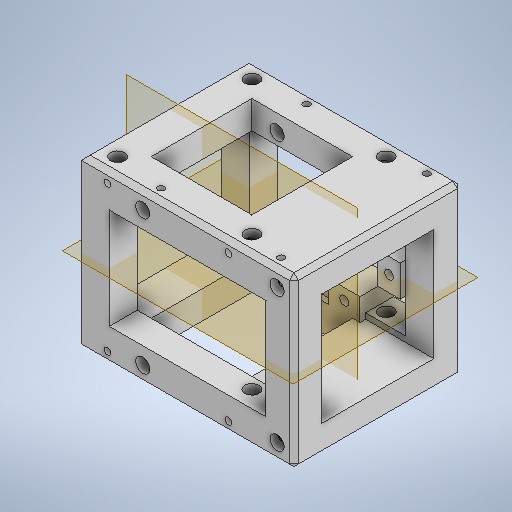
# Autodesk Inventor part: iluminator
Saved by Autodesk Inventor 2025.1 (Build 291241000, 241)
## iProperties
Created: 2024-11-24
Part Number: iluminator
Material: Ogólny
Document SubType Name: Modeling
Designer: zychlix
Density: 1 g/cm^3
Appearance: Domyślna
Author: zychlix
Autodesk Inventor part; units mm, degrees
ref_plane "YZ Plane" through (0, 0, 0) normal (1, 0, 0) x (0, 1, 0)
ref_plane "XZ Plane" through (0, 0, 0) normal (0, 1, 0) x (-1, 0, 0)
ref_plane "XY Plane" through (0, 0, 0) normal (0, 0, 1) x (1, 0, 0)
sketch "Szkic1" plane through (0, 0, 0) normal (0, 0, 1) x (1, 0, 0)
  line L0 (100.1486, 94.401) -> (40.1486, 94.401) construction
  line L1 (40.1486, 94.401) -> (40.1486, 34.401) construction
  line L2 (40.1486, 34.401) -> (100.1486, 34.401) construction
  line L3 (100.1486, 34.401) -> (100.1486, 94.401) construction
  circle A0 centre (100.1486, 94.401) radius 3.175
  circle A1 centre (100.1486, 34.401) radius 3.175
  circle A2 centre (40.1486, 34.401) radius 3.175
  circle A3 centre (40.1486, 94.401) radius 3.175
  line L4 (107.6486, 26.901) -> (12.6486, 26.901)
  line L5 (12.6486, 101.901) -> (107.6486, 101.901)
  line L6 (107.6486, 101.901) -> (107.6486, 26.901)
  line L7 (25.1486, 86.901) -> (95.1486, 86.901)
  line L8 (95.1486, 86.901) -> (95.1486, 41.901)
  line L9 (25.1486, 86.901) -> (25.1486, 41.901)
  line L10 (25.1486, 41.901) -> (95.1486, 41.901)
  line L11 (12.6486, 101.901) -> (12.6486, 26.901)
  point P0 (0, 0)
  point P1 (70.1486, 64.401)
  point P2 (100.1486, 64.401)
  point P3 (70.1486, 94.401)
  point P4 (107.6486, 64.401)
  point P5 (25.1486, 64.401)
  dimension "d0" = 60
  dimension "d1" = 60
  dimension "d2" = 6.35
  dimension "d8" = 75
  dimension "d39" = 7.5
  dimension "d40" = 5
  dimension "d61" = 45
  dimension "d63" = 12.5
  dimension "d64" = 95
  constraints: 24 end point, 4 centre point, 4 coincident, 4 midpoint, 4 parallel, 3 equal radius, 3 horizontal alignment, 3 perpendicular, 2 vertical, 1 horizontal, 1 vertical alignment
  measures "d0" distance of L2.end L0.start
  measures "d1" distance of L1.end L2.end
  measures "d2" diameter of A0
  measures "d8" distance of L5.end L4.start
  measures "d39" distance from line of L6 L0.start
  measures "d40" distance between parallel lines of L3 L8
  measures "d61" distance of L7.end L8.end
  measures "d63" distance between parallel lines of L11 L9
  measures "d64" distance between parallel lines of L6 L11
extrude "bryla" add sketch "Szkic1" against normal blind 75
sketch "Szkic2" plane through (12.6486, 101.901, 0) normal (0, 1, 0) x (1, 0, 0)
  line L0 (16.2355, 15) -> (16.2355, 60)
  circle A0 centre (68.7355, 67.5) radius 3.175
  line L1 (95, 0) -> (95, 75) projected
  line L2 (16.2355, 60) -> (61.2355, 60)
  line L3 (16.2355, 15) -> (61.2355, 15)
  line L4 (61.2355, 60) -> (61.2355, 15)
  line L5 (82.5, 0) -> (82.5, 75) projected
  circle A1 centre (68.7355, 67.5) radius 3 projected
  circle A2 centre (8.7355, 67.5) radius 3 projected
  circle A3 centre (8.7355, 7.5) radius 3 projected
  circle A4 centre (68.7355, 7.5) radius 3 projected
  circle A5 centre (68.7355, 7.5) radius 3.175
  circle A6 centre (8.7355, 7.5) radius 3.175
  circle A7 centre (8.7355, 67.5) radius 3.175
  line L6 (68.7355, 67.5) -> (8.7355, 67.5) construction
  line L7 (8.7355, 67.5) -> (8.7355, 7.5) construction
  point P0 (-12.6486, 0)
  point P1 (51.3842, 37.5)
  point P2 (51.3842, 53.4)
  point P3 (63.3142, 37.5)
  point P4 (38.7355, 67.5)
  point P5 (38.7355, 60)
  point P6 (8.7355, 37.5)
  point P7 (16.2355, 37.5)
  dimension "d32" = 6.35
  dimension "d65" = 45
  constraints: 12 end point, 4 centre point, 4 coincident, 4 midpoint, 3 equal radius, 3 horizontal, 2 horizontal alignment, 2 parallel, 2 perpendicular, 1 vertical alignment
  measures "d32" diameter of A0
  measures "d65" distance of L0.start L3.end
extrude "Wyciągnięcie proste2" cut sketch "Szkic2" against normal through all contours L0 L2 L4 L3 | A0 | A1 | A2 | A3 | A4 | A5 | A6 | A7
sketch "Szkic4" plane through (107.6486, 26.901, 0) normal (1, 0, 0) x (0, 0, -1)
  line L0 (0, 0) -> (0, 75) projected
  line L1 (0, 0) -> (75, 0) projected
  line L2 (75, 75) -> (75, 0) projected
  line L3 (0, 75) -> (75, 75) projected
  line L4 (12.5, 62.5) -> (12.5, 12.5)
  line L5 (12.5, 12.5) -> (62.5, 12.5)
  line L6 (62.5, 12.5) -> (62.5, 62.5)
  line L7 (62.5, 62.5) -> (12.5, 62.5)
  point P0 (0, -26.901)
  dimension "d17" = 12.5
  constraints: 8 end point, 3 other
  measures "d17" distance between parallel lines of L0 L4
extrude "Wyciągnięcie proste3" cut sketch "Szkic4" against normal through all contours L7 L6 L5 L4
sketch "Szkic5" plane through (0, 0, -75) normal (0, 0, -1) x (-1, 0, 0)
  line L0 (-77.1486, 39.401) -> (-63.1486, 39.401)
  line L1 (-63.1486, 39.401) -> (-63.1486, 49.401)
  line L2 (-63.1486, 49.401) -> (-77.1486, 49.401)
  line L3 (-77.1486, 49.401) -> (-77.1486, 39.401)
  line L4 (-77.1486, 79.401) -> (-63.1486, 79.401)
  line L5 (-63.1486, 79.401) -> (-63.1486, 86.901)
  line L6 (-63.1486, 86.901) -> (-77.1486, 86.901)
  line L7 (-77.1486, 86.901) -> (-77.1486, 79.401)
  line L8 (-55.1486, 57.401) -> (-31.2645, 57.401)
  line L9 (-31.2645, 57.401) -> (-31.2645, 71.401)
  line L10 (-31.2645, 71.401) -> (-55.1486, 71.401)
  line L11 (-55.1486, 71.401) -> (-55.1486, 57.401)
  line L12 (-31.2645, 39.401) -> (-95.1486, 39.401) construction
  line L13 (-31.2645, 86.901) -> (-31.2645, 39.401) construction
  line L14 (-95.1486, 86.901) -> (-25.1486, 86.901) construction
  circle A0 centre (-70.1486, 44.401) radius 2
  circle A1 centre (-50.1486, 64.401) radius 2
  circle A2 centre (-70.1486, 84.401) radius 2
  circle A3 centre (-90.1486, 64.401) radius 2
  line L15 (-95.1486, 86.901) -> (-95.1486, 41.901) projected
  line L16 (-85.1486, 57.401) -> (-95.1486, 57.401)
  line L17 (-95.1486, 57.401) -> (-95.1486, 71.401)
  line L18 (-95.1486, 71.401) -> (-85.1486, 71.401)
  line L19 (-85.1486, 71.401) -> (-85.1486, 57.401)
  point P0 (0, 0)
  point P1 (-70.1486, 64.401)
  point P2 (-55.1486, 64.401)
  point P3 (-70.1486, 49.401)
  point P4 (-70.1486, 79.401)
  point P5 (-90.1486, 71.401)
  point P6 (-90.1486, 57.401)
  point P7 (-95.1486, 57.401)
  dimension "d20" = 15
  dimension "d21" = 15
  dimension "d22" = 15
  dimension "d23" = 14
  dimension "d24" = 4
  dimension "d27" = 360
  dimension "d29" = 20
  dimension "d42" = 15
  constraints: 32 end point, 8 parallel, 5 collinear, 5 midpoint, 5 perpendicular, 4 centre point, 4 horizontal, 3 point on line, 2 vertical alignment, 1 horizontal alignment, 9 other
  measures "d20" distance from line of L2 point (-70.149, 64.401)
  measures "d21" distance from line of L4 point (-70.149, 64.401)
  measures "d22" distance from line of point (-70.149, 64.401) L11
  measures "d23" distance of L1.end L2.end
  measures "d24" diameter of A0
  measures "d29" distance of point (-70.149, 64.401) A0.centre
  measures "d42" distance from line of point (-70.149, 64.401) L19
extrude "Wyciągnięcie proste4" add sketch "Szkic5" against normal up to surface (15 mm away) contours L3 L2 L1 L0 | L7 L6 L5 L4 | L18 L19 L16 L15
ref_plane "Płaszczyzna konstrukcyjna1" through (12.6486, 64.401, 0) normal (0, 1, 0) x (1, 0, 0)
sketch "Szkic6" plane through (0, 0, 0) normal (0, 0, 1) x (1, 0, 0)
  circle A0 centre (78.3842, 96.901) radius 1.5
  circle A1 centre (24.3842, 96.901) radius 1.5
  line L0 (107.6486, 101.901) -> (12.6486, 101.901) projected
  circle A2 centre (78.3842, 31.901) radius 1.5
  circle A3 centre (24.3842, 31.901) radius 1.5
  line L1 (12.6486, 26.901) -> (107.6486, 26.901) projected
  line L2 (84.3842, 7.3) -> (84.3842, 507.3)
  line L3 (78.3842, 7.3) -> (78.3842, 507.3) construction
  line L4 (24.3842, 0) -> (24.3842, 500) construction
  point P0 (0, 0)
  dimension "d44" = 3
  dimension "d46" = 5
  dimension "d48" = 5
  constraints: 6 end point, 4 centre point, 3 equal radius, 3 point on line, 3 vertical, 2 horizontal alignment, 1 vertical alignment, 6 other
  measures "d44" diameter of A0
  measures "d46" distance from line of L0 A0.centre
  measures "d48" distance from line of L1 A3.centre
extrude "Wyciągnięcie proste5" cut sketch "Szkic6" against normal blind 10
sketch "Szkic9" plane through (12.6486, 26.901, 0) normal (0, -1, 0) x (1, 0, 0)
  line L0 (90.675, -75) -> (90.675, 0) projected
  line L1 (84.325, -75) -> (84.325, 0) projected
  line L2 (30.675, -15) -> (30.675, 0) projected
  line L3 (24.325, -15) -> (24.325, 0) projected
  circle A0 centre (84.325, -5) radius 1.5
  circle A1 centre (30.675, -5) radius 1.5
  line L4 (84.325, -75) -> (84.325, 0) projected
  circle A2 centre (84.325, -70) radius 1.5
  circle A3 centre (30.675, -70) radius 1.5
  point P0 (-12.6486, 0)
  dimension "d52" = 3
  dimension "d53" = 5
  dimension "d57" = 5
  constraints: 4 centre point, 3 equal radius, 3 point on line, 2 horizontal alignment, 2 vertical alignment
  measures "d52" diameter of A0
  measures "d53" distance of L1.end A0.centre
  measures "d57" distance of L1.start A2.centre
extrude "Wyciągnięcie proste6" cut sketch "Szkic9" against normal blind 10
mirror "Odbij2" about plane through (12.6486, 64.401, 0) normal (0, 1, 0) of "Wyciągnięcie proste6"
ref_plane "Płaszczyzna konstrukcyjna3" through (0, 0, -37.5) normal (0, 0, 1) x (1, 0, 0)
mirror "Odbij3" about plane through (0, 0, -37.5) normal (0, 0, 1) of "Wyciągnięcie proste5"
chamfer "Faza2" distance 2 angle 45 10 edges at (107.6486, 64.401, 0) (107.6486, 101.901, -37.5) (107.6486, 26.901, -37.5) (107.6486, 64.401, -75) (60.1486, 101.901, -75) (60.1486, 101.901, 0) (12.6486, 101.901, -37.5) (60.1486, 26.901, 0) (12.6486, 26.901, -37.5) (60.1486, 26.901, -75)
